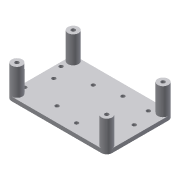
# Autodesk Inventor part: cellSTORM_v5_miniElectronics
Saved by Autodesk Inventor 2019.4 (Build 234330000, 330)
## iProperties
Created: 2020-06-15
Part Number: cellSTORM_v5_miniElectronics
Material: Generic
Document SubType Name: Modeling
Designer: diederichbenedict
Density: 1 g/cm^3
Appearance: White
Author: diederichbenedict
Autodesk Inventor part; units mm, degrees
ref_plane "YZ Plane" through (0, 0, 0) normal (1, 0, 0) x (0, 1, 0)
ref_plane "XZ Plane" through (0, 0, 0) normal (0, 1, 0) x (-1, 0, 0)
ref_plane "XY Plane" through (0, 0, 0) normal (0, 0, 1) x (1, 0, 0)
sketch "Sketch1" plane through (0, 0, 0) normal (0, 1, 0) x (-1, 0, 0)
  line L0 (37.5, 25) -> (-37.5, 25)
  line L1 (-37.5, 25) -> (-37.5, -25)
  line L2 (-37.5, -25) -> (37.5, -25)
  line L3 (37.5, -25) -> (37.5, 25)
  line L4 (37.5, 25) -> (-37.5, -25) construction
  line L5 (-37.5, 25) -> (37.5, -25) construction
  circle A0 centre (29.5, -0.5) radius 2 construction
  circle A1 centre (-30.5, -0.5) radius 2 construction
  circle A2 centre (29.5, -2.5) radius 1.45
  circle A3 centre (-30.5, -2.5) radius 1.45
  point P0 (0, 0)
  dimension "d0" = 75
  dimension "d1" = 50
  dimension "d9" = 2.9
  dimension "d10" = 2.9
  constraints: 12 end point, 2 centre point, 2 midpoint, 2 parallel, 2 vertical alignment, 1 horizontal, 1 perpendicular, 2 other
  measures "d0" distance of L2.end L1.end
  measures "d1" distance of L1.end L0.end
  measures "d9" diameter of A2
  measures "d10" diameter of A3
sketch "Sketch1 outline for Extrusion1" plane through (0, 0, 0) normal (0, 1, 0) x (-1, 0, 0)
  line L0 (37.5, -25) -> (37.5, 25)
  line L1 (-37.5, -25) -> (37.5, -25)
  line L2 (37.5, 25) -> (-37.5, 25)
  line L3 (-37.5, 25) -> (-37.5, -25)
  circle A0 centre (29.5, -2.5) radius 1.45
  circle A1 centre (-30.5, -2.5) radius 1.45
extrude "Extrusion1" add sketch "Sketch1 outline for Extrusion1" along normal blind 3
fillet "Fillet1" radius 4 4 edges at (-37.5, 1.5, 25) (37.5, 1.5, 25) (37.5, 1.5, -25) (-37.5, 1.5, -25)
sketch "Sketch2" plane through (0, 3, 0) normal (0, 1, 0) x (1, 0, 0)
  arc A0 (-33.5, 25) -> (-37.5, 21) centre (-33.5, 21) ccw projected
  line L0 (-37.5, 21) -> (-37.5, -21) projected
  arc A1 (-37.5, -21) -> (-33.5, -25) centre (-33.5, -21) ccw projected
  line L1 (-33.5, -25) -> (33.5, -25) projected
  arc A2 (33.5, -25) -> (37.5, -21) centre (33.5, -21) ccw projected
  line L2 (37.5, -21) -> (37.5, 21) projected
  arc A3 (37.5, 21) -> (33.5, 25) centre (33.5, 21) ccw projected
  line L3 (33.5, 25) -> (-33.5, 25) projected
  circle A4 centre (-33.5, -21) radius 4
  circle A5 centre (-33.5, 21) radius 4
  circle A6 centre (33.5, 21) radius 4
  circle A7 centre (33.5, -21) radius 4
  point P0 (0, 0)
  constraints: 4 centre point, 4 coincident, 4 concentric
sketch "Sketch2 outline for Extrusion2" plane through (0, 3, 0) normal (0, 1, 0) x (1, 0, 0)
  circle A0 centre (-33.5, -21) radius 4
  circle A1 centre (-33.5, 21) radius 4
  circle A2 centre (33.5, 21) radius 4
  circle A3 centre (33.5, -21) radius 4
extrude "Extrusion2" add sketch "Sketch2 outline for Extrusion2" along normal blind 20
sketch "Sketch3" plane through (-33.5, 23, -21) normal (0, 1, 0) x (1, 0, 0)
  circle A0 centre (0, 0) radius 4 projected
  circle A1 centre (67, 0) radius 4 projected
  circle A2 centre (67, -42) radius 4 projected
  circle A3 centre (0, -42) radius 4 projected
  point P0 (33.5, -21)
hole "Hole1" at (33.5, 23, -21) at (33.5, 23, 21) at (-33.5, 23, 21) at (-33.5, 23, -21) direction (0, -1, 0) diameter 3 end through all
sketch "Sketch4" plane through (0, 3, 0) normal (0, 1, 0) x (1, 0, 0)
  circle A0 centre (-34.514046, 12.932135) radius 1
  circle A1 centre (-10.514046, -14.067865) radius 1
  circle A2 centre (-34.514046, -14.067865) radius 1
  circle A3 centre (-34.514046, 12.932135) radius 1
  circle A4 centre (-10.514046, 12.932135) radius 1
  line L0 (-9.014046, -15.567865) -> (-9.014046, 14.432135)
  line L1 (-9.014046, 14.432135) -> (-36.014046, 14.432135)
  line L2 (-36.014046, 14.432135) -> (-36.014046, -15.567865)
  line L3 (-36.014046, -15.567865) -> (-9.014046, -15.567865)
  point P0 (0, 0)
hole "Hole2" at (-10.514046, 3, -12.932135) at (-10.514046, 3, 14.067865) at (-34.514046, 3, 14.067865) at (-34.514046, 3, -12.932135) direction (0, -1, 0) diameter 2.9 end through all
sketch "Sketch5" plane through (0, 3, 0) normal (0, 1, 0) x (1, 0, 0)
  circle A0 centre (29.048004, -12.336543) radius 0.5
  circle A1 centre (27.048004, -12.336543) radius 0.5
  circle A2 centre (25.048004, -12.336543) radius 0.5
  circle A3 centre (23.048004, -12.336543) radius 0.5
  circle A4 centre (21.048004, -12.336543) radius 0.5
  circle A5 centre (19.048004, -12.336543) radius 0.5
  circle A6 centre (17.048004, -12.336543) radius 0.5
  circle A7 centre (15.048004, -12.336543) radius 0.5
  circle A8 centre (13.048004, -12.336543) radius 0.5
  circle A9 centre (11.048004, -12.336543) radius 0.5
  circle A10 centre (29.048004, -14.336543) radius 0.5
  circle A11 centre (27.048004, -14.336543) radius 0.5
  circle A12 centre (25.048004, -14.336543) radius 0.5
  circle A13 centre (23.048004, -14.336543) radius 0.5
  circle A14 centre (21.048004, -14.336543) radius 0.5
  circle A15 centre (19.048004, -14.336543) radius 0.5
  circle A16 centre (17.048004, -14.336543) radius 0.5
  circle A17 centre (15.048004, -14.336543) radius 0.5
  circle A18 centre (13.048004, -14.336543) radius 0.5
  circle A19 centre (11.048004, -14.336543) radius 0.5
  line L0 (36.448004, 3.863457) -> (40.048004, 3.863457)
  line L1 (40.048004, 3.863457) -> (40.048004, 4.163457)
  line L2 (40.048004, 4.163457) -> (42.048004, 4.163457)
  line L3 (42.048004, 4.163457) -> (42.048004, 15.163457)
  line L4 (42.048004, 15.163457) -> (5.048004, 15.163457)
  line L5 (5.048004, 15.163457) -> (3.048004, 13.163457)
  line L6 (3.048004, 13.163457) -> (3.048004, -14.036543)
  line L7 (3.048004, -14.036543) -> (5.048004, -16.036543)
  line L8 (5.048004, -16.036543) -> (35.748004, -16.036543)
  line L9 (35.748004, -16.036543) -> (35.748004, -13.436543)
  line L10 (35.748004, -13.436543) -> (36.448004, -13.436543)
  line L11 (36.448004, -13.436543) -> (36.448004, -11.381199)
  line L12 (36.448004, -11.381199) -> (41.474904, -11.381199)
  line L13 (41.474904, -11.381199) -> (41.474904, -13.436543)
  line L14 (41.474904, -13.436543) -> (42.048004, -13.436543)
  line L15 (42.048004, -13.436543) -> (42.048004, -5.136543)
  line L16 (42.048004, -5.136543) -> (40.048004, -5.136543)
  line L17 (40.048004, -5.136543) -> (40.048004, -4.336543)
  line L18 (40.048004, -4.336543) -> (36.448004, -4.336543)
  line L19 (36.448004, -4.336543) -> (36.448004, 3.863457)
  line L20 (10.248004, -8.436543) -> (10.248004, 7.063457)
  line L21 (10.248004, 7.063457) -> (27.748004, 7.063457)
  line L22 (27.748004, 7.063457) -> (27.748004, -8.436543)
  line L23 (27.748004, -8.436543) -> (10.248004, -8.436543)
  circle A20 centre (27.048004, -17.806741) radius 1.45
  circle A21 centre (7.806396, -17.806741) radius 1.45
  circle A22 centre (7.806396, 16.763599) radius 1.45
  circle A23 centre (26.781094, 16.763599) radius 1.45
  point P0 (0, 0)
  dimension "d25" = 2.9
  dimension "d26" = 2.9
  dimension "d27" = 2.9
  dimension "d28" = 2.9
  constraints: 4 centre point
  measures "d25" diameter of A20
  measures "d26" diameter of A21
  measures "d27" diameter of A22
  measures "d28" diameter of A23
sketch "Sketch5 outline for Extrusion3" plane through (0, 3, 0) normal (0, 1, 0) x (1, 0, 0)
  circle A0 centre (27.048004, -17.806741) radius 1.45
  circle A1 centre (7.806396, -17.806741) radius 1.45
  circle A2 centre (7.806396, 16.763599) radius 1.45
  circle A3 centre (26.781094, 16.763599) radius 1.45
extrude "Extrusion3" cut sketch "Sketch5 outline for Extrusion3" against normal blind 15
body "Solid1"
